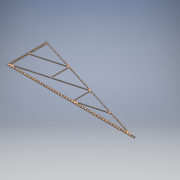
# Autodesk Inventor part: side
Saved by Autodesk Inventor 2018.3 (Build 223284000, 284)
## iProperties
Created: 2018-05-24
Part Number: side
Material: Wood (Birch)
Document SubType Name: Modeling
Designer: mzhang
Density: 0.55 g/cm^3
Appearance: Birch - Natural Polished
Mass: 4.00431 g
Surface Area: 147.823 cm^2
Volume: 7.28056 cm^3
Author: mzhang
Autodesk Inventor part; units mm, degrees
ref_plane "YZ Plane" through (0, 0, 0) normal (1, 0, 0) x (0, 1, 0)
ref_plane "XZ Plane" through (0, 0, 0) normal (0, 1, 0) x (-1, 0, 0)
ref_plane "XY Plane" through (0, 0, 0) normal (0, 0, 1) x (1, 0, 0)
sketch "Sketch1" plane through (0, 0, 0) normal (0, 0, 1) x (1, 0, 0)
  line L0 (0, 0) -> (481, 0)
  line L1 (481, 0) -> (481, 150)
  line L2 (0, 150) -> (0, 0)
  line L3 (481, 0) -> (5.5984, 148.2541)
  line L4 (0, 0) -> (481, 0)
  line L5 (0, 6) -> (0, 0)
  line L6 (455.0421, 6) -> (0, 6)
  line L7 (7.4878, 6) -> (241.4514, 70.8476)
  line L8 (241.4514, 70.8476) -> (244.4407, 71.6761)
  line L9 (455.0421, 6) -> (244.4407, 71.6761)
  line L10 (5.5984, 146.1591) -> (5.5984, 7.5517)
  line L11 (5.5984, 146.1591) -> (144.2058, 146.1591) construction
  line L12 (8, 145.4102) -> (7.4878, 8.0754)
  line L13 (0, 6) -> (5.5984, 7.5517)
  line L14 (7.4878, 8.0754) -> (240.9172, 72.7749)
  line L15 (240.9172, 72.7749) -> (8, 145.4102)
  line L16 (5.5984, 146.1591) -> (0, 146.1591)
  line L17 (5.5984, 148.2541) -> (0, 148.2541)
  point P0 (0, 147.905)
  dimension "d4" = 250
  dimension "d7" = 90
  constraints: 36 end point, 6 parallel, 4 perpendicular, 4 point on line, 3 horizontal
  measures "d4" distance of L5.start L14.end
  measures "d7" angle of L10 L11
extrude "Extrusion1" add sketch "Sketch1" along normal blind 1.5875 contours L2 L13 L10 L16 L17 L3 L0
sketch "Sketch2" plane through (0, 0, 1.5875) normal (0, 0, 1) x (1, 0, 0)
  line L0 (11, 2.2063) -> (6, 2.2063)
  line L1 (6, 2.2063) -> (6, 3.7937)
  line L2 (6, 3.7937) -> (11, 3.7938)
  line L3 (11, 3.7938) -> (11, 2.2063)
  line L4 (11, 2.2063) -> (6, 3.7937) construction
  line L5 (6, 2.2063) -> (11, 3.7938) construction
  line L6 (0, 6) -> (0, 0) projected
  line L7 (0, 0) -> (481, 0) projected
  point P0 (8.5, 3)
  dimension "d10" = 1.5875
  dimension "d11" = 6
  dimension "d12" = 3
  dimension "d15" = 5
  constraints: 12 end point, 2 midpoint, 2 parallel, 1 horizontal, 1 perpendicular
  measures "d10" distance of L0.end L1.end
  measures "d11" distance between parallel lines of L6 L1
  measures "d12" distance from line of L7 point (8.5, 3)
  measures "d15" distance of L0.start L0.end
extrude "Extrusion2" cut sketch "Sketch2" against normal blind 1.5875
pattern_linear "Rectangular Pattern1" count 48 spacing 10 along (1, 0, 0) of "Extrusion2"
sketch "Sketch3" plane through (0, 0, 1.5875) normal (0, 0, 1) x (1, 0, 0)
  line L0 (5.5984, 146.1591) -> (5.5984, 7.5517) projected
  line L1 (5.5984, 143.1591) -> (0, 143.1591)
  line L2 (0, 143.1591) -> (0, 140.1591)
  line L3 (0, 140.1591) -> (5.5984, 140.1591)
  line L4 (5.5984, 140.1591) -> (5.5984, 143.1591)
  point P0 (0, 0)
  dimension "d19" = 3
  dimension "d20" = 3
  constraints: 8 end point, 2 parallel, 1 horizontal, 1 perpendicular, 1 point on line
  measures "d19" distance of L2.end L1.end
  measures "d20" distance from line of L1 L0.start
extrude "Extrusion3" add sketch "Sketch3" against normal blind 1.5875
sketch "Sketch4" plane through (0, 0, 1.5875) normal (0, 0, 1) x (1, 0, 0)
  line L0 (5.5984, 7.5517) -> (0, 6) projected
  line L1 (1.2436, 6.3447) -> (193.6502, 6.3447) construction
  line L2 (0, 0) -> (481, 0) projected
  line L3 (1.5875, -0.8087) -> (204.2972, -0.8087) construction
  line L4 (5.5984, 148.2541) -> (0, 148.2541) projected
  line L5 (5.5984, 143.1591) -> (0, 143.1591) projected
  line L6 (0, 146.1591) -> (5.5984, 146.1591) projected
  line L7 (0, 140.1591) -> (5.5984, 140.1591) projected
  line L8 (1.5875, 6.44) -> (1.5875, 140.1591)
  line L9 (1.5875, 143.1591) -> (1.5875, 146.1591)
  line L10 (3.5875, 148.2541) -> (3.5875, 6.9943)
  line L11 (3.5875, 148.2541) -> (144.8473, 148.2541) construction
  line L12 (1.5875, 6.44) -> (3.5875, 6.9943)
  line L13 (1.5875, 148.2541) -> (1.5875, 146.1591)
  line L14 (1.5875, 143.1591) -> (1.5875, 140.1591)
  line L15 (1.5875, 148.2541) -> (3.5875, 148.2541)
  point P0 (1.5875, 0)
  dimension "d25" = 90
  constraints: 20 end point, 9 point on line, 3 horizontal, 3 perpendicular, 2 collinear
  measures "d25" angle of L10 L11
extrude "Extrusion4" add sketch "Sketch4" against normal blind 1.5875
fillet "Fillet1" radius 2 6 edges at (8, 145.4102, 0.7937) (244.4407, 71.6761, 0.7937) (240.9172, 72.7749, 0.7937) (455.0421, 6, 0.7937) (7.4878, 8.0754, 0.7937) (7.4878, 6, 0.7937)
sketch "Sketch5" plane through (0, 0, 1.5875) normal (0, 0, 1) x (1, 0, 0)
  line L0 (0, 0) -> (481, 0) projected
  line L1 (468.8347, 3.7938) -> (5.5984, 148.2541) projected
  line L2 (464.7971, 5.0529) -> (481, 5.0529)
  line L3 (481, 5.0529) -> (481, 0)
  line L4 (461, 3.7938) -> (456, 3.7937) projected
  line L5 (461, 2.2063) -> (461, 3.7938) projected
  line L6 (456, 2.2063) -> (461, 2.2063)
  line L7 (461, 2.2063) -> (461, 3.7938)
  line L8 (461, 3.7938) -> (456, 3.7938)
  line L9 (456, 3.7938) -> (456, 2.2063)
  line L10 (456, 2.2063) -> (461, 3.7938) construction
  line L11 (461, 2.2063) -> (456, 3.7938) construction
  line L12 (471, 3.7938) -> (466, 3.7938)
  line L13 (471, 2.2063) -> (471, 3.7938)
  line L14 (466, 2.2063) -> (471, 2.2063)
  line L15 (466, 3.7938) -> (466, 2.2063)
  line L16 (481, 3.7938) -> (476, 3.7938)
  line L17 (481, 2.2063) -> (481, 3.7938)
  line L18 (476, 2.2063) -> (481, 2.2063)
  line L19 (476, 3.7938) -> (476, 2.2063)
  line L20 (471, 2.2063) -> (471, 3.1185) projected
  line L21 (481, 0) -> (471, 3.1185) projected
  line L22 (471, 3.1185) -> (481, 0)
  line L23 (468.8347, 3.7938) -> (471, 3.7938)
  point P0 (458.5, 3.7938)
  point P1 (461, 3)
  point P2 (458.5, 3)
  dimension "d31" = 10
  constraints: 36 end point, 4 midpoint, 3 horizontal, 2 collinear, 2 parallel, 2 perpendicular, 1 point on line, 16 other
  measures "d31" distance of L4.start L12.start
extrude "Extrusion5" add sketch "Sketch5" against normal up to surface (1.5875 mm away) contours L1 L2 L3 L16 L19 L18 L21 L13 L12
fillet "Fillet2" radius 1 2 edges at (481, 0, 0.7937) (481, 5.0529, 0.7937)
sketch "Sketch6" plane through (0, 0, 1.5875) normal (0, 0, 1) x (1, 0, 0)
  line L0 (245.4394, 71.3647) -> (245.4394, 6)
  line L1 (243.4394, 71.3985) -> (243.4394, 6)
  line L2 (243.4394, 71.3985) -> (243.8733, 71.5188)
  arc A0 (245.0029, 71.5008) -> (243.8733, 71.5188) centre (244.4075, 69.5915) ccw projected
  arc A1 (245.0029, 71.5008) -> (243.8733, 71.5188) centre (244.4075, 69.5915) ccw
  line L3 (245.0029, 71.5008) -> (245.4394, 71.3647)
  line L4 (243.4394, 6) -> (245.4394, 6)
  point P0 (0, 0)
  constraints: 10 end point, 2 point on circle, 1 centre point, 1 perpendicular
extrude "Extrusion6" add sketch "Sketch6" against normal blind 1.5875
fillet "Fillet3" radius 4 4 edges at (243.4394, 71.3985, 0.7937) (245.4394, 71.3647, 0.7937) (243.4394, 6, 0.7937) (245.4394, 6, 0.7937)
sketch "Sketch7" plane through (0, 0, 1.5875) normal (0, 0, 1) x (1, 0, 0)
  line L0 (245.4394, 10) -> (245.4394, 65.9273) projected
  line L1 (249.4394, 6) -> (441.9108, 6) projected
  line L2 (245.4394, 18.8313) -> (259.2517, 18.8313)
  line L3 (259.2517, 18.8313) -> (259.2517, 6)
  line L4 (259.2517, 6) -> (245.4394, 6)
  line L5 (245.4394, 6) -> (245.4394, 18.8313)
  point P0 (0, 0)
  constraints: 8 end point, 2 parallel, 2 point on line, 1 horizontal, 1 perpendicular
extrude "Extrusion7" cut sketch "Sketch7" against normal blind 1.5875
sketch "Sketch8" plane through (0, 0, 1.5875) normal (0, 0, 1) x (1, 0, 0)
  line L0 (441.9108, 6) -> (245.4394, 6) projected
  line L1 (21.6573, 9.9273) -> (238.371, 69.9937) projected
  line L2 (354.6496, 37.3074) -> (245.4394, 7.0377)
  line L3 (356.6784, 35.7944) -> (252.7912, 7)
  line L4 (252.7912, 7) -> (249.1833, 6)
  line L5 (250.6302, 69.7459) -> (442.5062, 9.9093) projected
  line L6 (356.6784, 35.7944) -> (358.173, 36.2086)
  line L7 (245.4394, 6) -> (245.4394, 65.9273) projected
  point P0 (0, 0)
  constraints: 8 end point, 3 point on line
extrude "Extrusion8" add sketch "Sketch8" against normal blind 1.5875
fillet "Fillet4" radius 3 2 edges at (245.4394, 7.0377, 0.7937) (354.6496, 37.3074, 0.7937)
fillet "Fillet5" radius 2 1 edges at (249.1833, 6, 0.7937)
sketch "Sketch9" plane through (0, 0, 1.5875) normal (0, 0, 1) x (1, 0, 0)
  line L0 (7.7477, 77.7475) -> (122.7547, 109.6239)
  line L1 (8.0109, 75.7451) -> (124.7835, 108.1109)
  line L2 (8.0109, 75.7451) -> (7.7399, 75.6699)
  line L3 (124.7835, 108.1109) -> (126.2782, 108.5251)
  line L4 (7.7477, 77.7475) -> (7.7399, 75.6699)
  line L5 (122.7547, 109.6239) -> (126.2782, 108.5251)
  point P0 (0, 0)
  constraints: 12 end point
extrude "Extrusion9" add sketch "Sketch9" against normal blind 1.5875
fillet "Fillet6" radius 4 2 edges at (7.7399, 75.6699, 0.7937) (7.7477, 77.7475, 0.7937)
fillet "Fillet7" radius 2 1 edges at (122.7547, 109.6239, 0.7937)
sketch "Sketch10" plane through (0, 0, 0) normal (0, 0, -1) x (-1, 0, 0)
  line L0 (-126.2782, 108.5251) -> (-234.4324, 74.7972) projected
  line L1 (-234.3712, 70.9605) -> (-10.0319, 8.7805) projected
  line L2 (-127.2782, 41.2776) -> (-127.2782, 107.1658)
  line L3 (-125.2782, 41.0004) -> (-125.2782, 108.248)
  line L4 (-125.2782, 41.0004) -> (-125.2782, 40.7233)
  line L5 (-126.2782, 108.5251) -> (-10.6602, 76.4794) projected
  line L6 (-127.2782, 107.1658) -> (-127.2782, 108.2133)
  point P0 (0, 0)
  constraints: 8 end point, 4 point on line, 2 vertical
extrude "Extrusion10" add sketch "Sketch10" against normal blind 1.5875
fillet "Fillet8" radius 4 3 edges at (125.2782, 40.7233, 0.7937) (127.2782, 41.2776, 0.7937) (125.2782, 108.248, 0.7937)
fillet "Fillet9" radius 3 1 edges at (127.2782, 108.2133, 0.7937)
body "Solid1"
